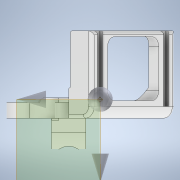
# Autodesk Inventor part: franka_connector
Saved by Autodesk Inventor 2022 (Build 260153000, 153)
## iProperties
Created: 2021-06-02
Part Number: franka_connector
Material: ABS Plastic
Document SubType Name: Modeling
Designer: fraaw
Density: 1.06 g/cm^3
Appearance: Smooth - White
Mass: 33.0638 g
Surface Area: 153.412 cm^2
Volume: 31.1922 cm^3
Author: fraaw
## iProperties of the stored document franka_connector_3DPrint.ipt
Created: 2021-06-08
Part Number: franka_connector_3DPrint
Material: Generic
Document SubType Name: Modeling
Designer: fraaw
Density: 1 g/cm^3
Appearance: Default
Author: fraaw
Autodesk Inventor part; units mm, degrees
note: some values were not read from the file. Chosen so that the rebuilt part matches the saved one: direction of "Hole1".
ref_plane "YZ Plane" through (0, 0, 0) normal (1, 0, 0) x (0, 1, 0)
ref_plane "XZ Plane" through (0, 0, 0) normal (0, 1, 0) x (-1, 0, 0)
ref_plane "XY Plane" through (0, 0, 0) normal (0, 0, 1) x (1, 0, 0)
sketch "Sketch1" plane through (0, 0, 0) normal (0, 1, 0) x (-1, 0, 0)
  line L0 (5, 5) -> (-5, 5) construction
  line L1 (-5, 5) -> (-5, -5) construction
  line L2 (-5, -5) -> (5, -5) construction
  line L3 (5, -5) -> (5, 5) construction
  line L4 (5, 5) -> (-5, -5) construction
  line L5 (-5, 5) -> (5, -5) construction
  line L6 (5, -5) -> (-5, -5) construction
  line L7 (-5, -5) -> (-5, -25)
  line L8 (-5, -25) -> (5, -25)
  line L9 (5, -25) -> (5, -5)
  line L10 (25, 5) -> (5, 5)
  line L11 (25, -5) -> (25, 5)
  line L12 (5, -5) -> (25, -5)
  line L13 (-5, 25) -> (-5, 5)
  line L14 (5, 25) -> (-5, 25)
  line L15 (5, 5) -> (5, 25)
  line L16 (-25, -5) -> (-5, -5)
  line L17 (-25, 5) -> (-25, -5)
  line L18 (-5, 5) -> (-25, 5)
  point P0 (0, 0)
  point P1 (5, -5)
  dimension "d7" = 10
  dimension "d8" = 10
  dimension "d9" = 20
  dimension "d12" = 360
  constraints: 38 end point, 5 equal length, 2 midpoint, 2 perpendicular, 1 horizontal, 29 other
  measures "d7" distance of L1.end L2.end
  measures "d8" distance of L2.end L0.start
  measures "d9" distance of L8.end L2.end
extrude "Extrusion1" add sketch "Sketch1" along normal blind 8
sketch "Sketch2" plane through (0, 8, 0) normal (0, 1, 0) x (1, 0, 0)
  line L0 (5, 25) -> (-5, 25) projected
  circle A0 centre (0, 25) radius 7
  circle A1 centre (-25, 0) radius 7
  circle A2 centre (0, -25) radius 7
  circle A3 centre (25, 0) radius 7
  point P0 (0, 0)
  dimension "d16" = 14
  dimension "d19" = 360
  constraints: 4 centre point, 1 midpoint, 9 other
  measures "d16" diameter of A0
extrude "Base Holes" add sketch "Sketch2" against normal up to surface (8 mm away)
sketch "Sketch3" plane through (0, 8, 0) normal (0, 1, 0) x (1, 0, 0)
  arc A0 (-20.101, 5) -> (-20.101, -5) centre (-25, 0) ccw projected
  point P0 (0, 0)
  point P1 (0, -25)
  point P2 (25, 0)
  point P3 (0, 25)
  dimension "d33" = 360
  constraints: 1 coincident, 5 other
hole "Hole1" at (-25, 8, 0) at (0, 8, 25) at (25, 8, 0) at (0, 8, -25) direction (0, -1, 0) diameter 6.2 depth 8 counterbore diameter 10.1 counterbore depth 4
sketch "Sketch4" plane through (0, 0, 0) normal (0, -1, 0) x (1, 0, 0)
  circle A0 centre (0, -25) radius 3.1 projected
  arc A1 (-5, -20.101) -> (5, -20.101) centre (0, -25) ccw projected
  arc A2 (-5, -20.101) -> (0, -32) centre (0, -25) ccw
  circle A3 centre (-25, 0) radius 3.1 projected
  arc A4 (-20.101, 5) -> (-20.101, -5) centre (-25, 0) ccw projected
  arc A5 (-32, 0) -> (-20.101, -5) centre (-25, 0) ccw
  line L0 (-5, -20.101) -> (-5, -5) projected
  line L1 (-5, -20.101) -> (-5, -5)
  line L2 (-5, -5) -> (-20.101, -5)
  line L3 (-32, 0) -> (-43.1335, 0)
  line L4 (-52.6795, -9.5459) -> (-9.5459, -52.6795)
  line L5 (0, -43.1335) -> (0, -32)
  circle A6 centre (0, 0) radius 44 construction
  line L6 (-43.1335, 0) -> (-52.6795, -9.5459)
  line L7 (-9.5459, -52.6795) -> (0, -43.1335)
  dimension "d49" = 88
  dimension "d50" = 61
  constraints: 14 end point, 8 point on circle, 3 centre point, 3 coincident, 3 perpendicular, 2 equal length, 1 collinear, 1 horizontal, 1 tangent, 1 vertical
  measures "d49" diameter of A6
  measures "d50" distance of L4.start L4.end
extrude "Extrusion3" add sketch "Sketch4" against normal up to surface (8 mm away) contours A1 L5 L7 L4 L6 L3 A4 L2 L0
sketch "Sketch5" plane through (0, 8, 0) normal (0, 1, 0) x (1, 0, 0)
  point P0 (0, 0)
sketch "Sketch6" plane through (0, 8, 0) normal (0, 1, 0) x (1, 0, 0)
  line L0 (-52.6795, 9.5459) -> (-9.5459, 52.6795) projected
  line L1 (-52.6795, 9.5459) -> (-9.5459, 52.6795)
  line L2 (-9.5459, 52.6795) -> (-11.6673, 54.8008)
  line L3 (-11.6673, 54.8008) -> (-54.8008, 11.6673)
  line L4 (-54.8008, 11.6673) -> (-52.6795, 9.5459)
  point P0 (0, 0)
  dimension "d54" = 3
  constraints: 8 end point, 3 equal length, 1 perpendicular
  measures "d54" distance of L3.end L0.start
extrude "Extrusion4" add sketch "Sketch6" against normal blind 45
sketch "Skecth7" plane through (0, 0, 0) normal (0, -1, 0) x (1, 0, 0)
  line L0 (-43.1335, 0) -> (-52.6795, -9.5459) projected
  arc A0 (-43.9916, -0.8581) -> (-0.8581, -43.9916) centre (0, 0) ccw
  line L1 (-9.5459, -52.6795) -> (0, -43.1335) projected
  line L2 (-43.9916, -0.8581) -> (-52.6795, -9.5459)
  line L3 (-43.1335, 0) -> (-54.8008, -11.6673) projected
  line L4 (-52.6795, -9.5459) -> (-9.5459, -52.6795) projected
  line L5 (-31.1127, -31.1127) -> (-9.5459, -52.6795)
  line L6 (-9.5459, -52.6795) -> (-0.8581, -43.9916)
  point P0 (-31.1127, -31.1127)
  dimension "d57" = 44
  constraints: 6 end point, 2 collinear, 2 point on circle, 2 point on line, 1 centre point, 1 coincident, 1 midpoint, 1 perpendicular
  measures "d57" radius of A0
extrude "Extrusion5" add sketch "Skecth7" along normal up to surface (37 mm away)
sketch "Sketch8" plane through (0, -37, 0) normal (0, -1, 0) x (1, 0, 0)
  line L0 (-54.8008, -11.6673) -> (-11.6673, -54.8008) projected
  line L1 (0, 0) -> (-33.234, -33.234) construction
  line L2 (-11.6673, -54.8008) -> (-54.8008, -11.6673) projected
  line L3 (-50.2046, -16.2635) -> (-47.3762, -13.435) construction
  line L4 (-50.2046, -16.2635) -> (-51.6188, -14.8492)
  line L5 (-49.851, -10.9602) -> (-47.3762, -13.435)
  line L6 (-51.6188, -14.8492) -> (-49.851, -10.9602)
  line L7 (-50.2046, -16.2635) -> (-48.7904, -17.6777)
  line L8 (-44.9013, -15.9099) -> (-47.3762, -13.435)
  line L9 (-48.7904, -17.6777) -> (-44.9013, -15.9099)
  line L10 (-16.2635, -50.2046) -> (-13.435, -47.3762) construction
  line L11 (-16.2635, -50.2046) -> (-14.8492, -51.6188)
  line L12 (-10.9602, -49.851) -> (-13.435, -47.3762)
  line L13 (-14.8492, -51.6188) -> (-10.9602, -49.851)
  line L14 (-15.9099, -44.9013) -> (-13.435, -47.3762)
  line L15 (-17.6777, -48.7904) -> (-15.9099, -44.9013)
  line L16 (-16.2635, -50.2046) -> (-17.6777, -48.7904)
  dimension "d81" = 24
  dimension "d82" = 4
  dimension "d83" = 3.5
  dimension "d86" = 2
  constraints: 30 end point, 8 symmetric about line, 3 perpendicular, 2 point on line, 1 midpoint
  measures "d81" distance between parallel lines of L3 L1
  measures "d82" distance from line of L3.end L0
  measures "d83" distance of L5.start L3.end
  measures "d86" distance of L3.start L4.end
extrude "Extrusion6" cut sketch "Sketch8" against normal blind 39
sketch "Sketch18" plane through (0, 8, 0) normal (0, 1, 0) x (1, 0, 0)
  line L0 (8.8, -8.8) -> (-8.8, -8.8)
  line L1 (-8.8, -8.8) -> (-8.8, 8.8)
  line L2 (-8.8, 8.8) -> (8.8, 8.8)
  line L3 (8.8, 8.8) -> (8.8, -8.8)
  line L4 (8.8, -8.8) -> (-8.8, 8.8) construction
  line L5 (-8.8, -8.8) -> (8.8, 8.8) construction
  point P0 (0, 0)
  dimension "d89" = 17.6
  dimension "d90" = 17.6
  constraints: 12 end point, 2 midpoint, 2 parallel, 1 horizontal, 1 perpendicular
  measures "d89" distance of L0.end L1.end
  measures "d90" distance of L1.end L2.end
extrude "Rotator" add sketch "Sketch18" along normal blind 16
fillet "Fillet1" radius 8.8 2 edges at (8.8, 24, 0) (-8.8, 24, 0)
sketch "Sketch9" plane through (8.8, 8, -8.8) normal (0, 0, -1) x (-1, 0, 0)
  arc A0 (17.6, 7.2) -> (0, 7.2) centre (8.8, 7.2) ccw projected
  circle A1 centre (8.8, 7.2) radius 2.4
  point P0 (8.8, -8)
  dimension "d94" = 4.8
  constraints: 1 centre point, 1 coincident
  measures "d94" diameter of A1
extrude "Extrusion8" cut sketch "Sketch9" against normal up to next
sketch "Sketch10" plane through (0, 0, 0) normal (0, -1, 0) x (1, 0, 0)
  line L0 (5, 5) -> (20.101, 5) projected
  arc A0 (14.8825, -5) -> (14.8825, 5) centre (0, 0) ccw
  line L1 (20.101, -5) -> (5, -5) projected
  line L2 (14.8825, 5) -> (5, 5)
  line L3 (5, -5) -> (5, -8.8) projected
  line L4 (14.8825, -5) -> (5, -5)
  arc A1 (5, 14.8825) -> (-5, 14.8825) centre (0, 0) ccw
  line L5 (-5, 14.8825) -> (-5, 5)
  line L6 (5, 14.8825) -> (5, 5)
  arc A2 (-14.8825, 5) -> (-14.8825, -5) centre (0, 0) ccw
  line L7 (-14.8825, -5) -> (-5, -5)
  line L8 (-14.8825, 5) -> (-5, 5)
  arc A3 (-5, -14.8825) -> (5, -14.8825) centre (0, 0) ccw
  line L9 (5, -14.8825) -> (5, -5)
  line L10 (-5, -14.8825) -> (-5, -5)
  dimension "d97" = 15.7
  dimension "d100" = 360
  constraints: 16 end point, 8 point on circle, 4 centre point, 2 point on line, 1 coincident, 1 collinear, 1 horizontal, 33 other
  measures "d97" radius of A0
extrude "Extrusion9" add sketch "Sketch10" along normal blind 2.5
sketch "Sketch21" plane through (0, -2.5, 0) normal (0, -1, 0) x (1, 0, 0)
  circle A0 centre (0, 0) radius 5
  dimension "d104" = 10
  constraints: 1 centre point, 1 coincident
  measures "d104" diameter of A0
extrude "Extrusion10" cut sketch "Sketch21" against normal up to next
chamfer "Chamfer1" distance 8 angle 45 1 edges at (-31.1127, 0, -31.1127)
sketch "Sketch22" plane through (-54.8008, -37, -11.6673) normal (-0.7071068, 0, -0.7071068) x (-0.7071068, 0, 0.7071068)
  line L0 (-8.5, 0) -> (-52.5, 0) projected
  line L1 (-52.5, 39) -> (-51, 39) projected
  line L2 (-8.5, 0) -> (-52.5, 39) construction
  line L3 (-52.5, 0) -> (-8.5, 39) construction
  line L4 (-11.8846, 36) -> (-49.1154, 36)
  line L5 (-49.1154, 36) -> (-49.1154, 3)
  line L6 (-49.1154, 3) -> (-11.8846, 3)
  line L7 (-11.8846, 3) -> (-11.8846, 36)
  line L8 (-11.8846, 36) -> (-49.1154, 3) construction
  line L9 (-49.1154, 36) -> (-11.8846, 3) construction
  point P0 (-30.5, 37)
  point P1 (-30.5, 19.5)
  dimension "d107" = 3
  constraints: 16 end point, 3 midpoint, 3 point on line, 2 parallel, 1 horizontal, 1 perpendicular
  measures "d107" distance between parallel lines of L6 L0
extrude "Extrusion11" cut sketch "Sketch22" against normal up to next
fillet "Fillet3" radius 2.5 4 edges at (0, -2.5, 15.7) (-15.7, -2.5, 0) (0, -2.5, -15.7) (15.7, -2.5, 0)
fillet "Fillet4" radius 5 4 edges at (-14.7592, -1, -41.0853) (-41.0853, -1, -14.7592) (-43.8756, -34, -17.5495) (-17.5495, -34, -43.8756)
sketch "Sketch23" plane through (0, 0, 0) normal (0, 0, 1) x (1, 0, 0)
  line L0 (0, 0) -> (0, -7.1335) projected
  line L1 (0, -7.1335) -> (0, 8) projected
  ellipse E0 centre (0, -20) end of major axis (0, -30) minor radius 7.5
  line L2 (0, 0) -> (7, 0) projected
  point P0 (5, 0)
  dimension "d148" = 10
  dimension "d149" = 7.5
  dimension "d147" = 20
  constraints: 1 point on line, 2 other
  measures "d147" distance from line of L2 point (0, -20)
extrude "Extrusion12" cut sketch "Sketch23" against normal up to next
fillet "Fillet5" radius 6 1 edges at (-33.234, 8, -33.234)
sketch "Sketch28" plane through (0, 8, 0) normal (0, 1, 0) x (1, 0, 0)
  line L0 (-8.8, 8.8) -> (5, 8.8) projected
  line L1 (-8.8, 8.8) -> (-28.9914, 28.9914) construction
  line L2 (-50.5581, 7.4246) -> (-7.4246, 50.5581) projected
  line L3 (-16.2635, 19.0919) -> (-23.3345, 26.163)
  line L4 (-23.3345, 26.163) -> (-26.163, 23.3345)
  line L5 (-26.163, 23.3345) -> (-19.0919, 16.2635)
  line L6 (-19.0919, 16.2635) -> (-16.2635, 19.0919)
  line L7 (-16.2635, 19.0919) -> (-26.163, 23.3345) construction
  line L8 (-23.3345, 26.163) -> (-19.0919, 16.2635) construction
  point P0 (0, 0)
  point P1 (-21.2132, 21.2132)
  dimension "d141" = 10
  dimension "d143" = 4
  dimension "d144" = 11
  constraints: 14 end point, 3 midpoint, 2 parallel, 2 perpendicular, 1 point on line
  measures "d141" distance of L4.end L5.end
  measures "d143" distance of L3.end L4.end
  measures "d144" distance from line of L2 point (-21.213, 21.213)
extrude "Extrusion16" cut sketch "Sketch28" against normal up to next
fillet "Fillet6" radius 2 9 edges at (-53.5582, 6.2427, -10.4246) (-46.8459, 8, -3.7123) (-54.8008, -17.5, -11.6673) (-10.4246, 6.2427, -53.5582) (-3.7123, 8, -46.8459) (-11.6673, -17.5, -54.8008) (-33.234, -37, -33.234) (-53.2098, -37, -13.2583) (-13.2583, -37, -53.2098)
fillet "Fillet7" radius 1 6 edges at (6.9, 8, 8.8) (8.8, 8, 6.9) (-6.9, 8, 8.8) (-8.8, 8, 6.9) (6.9, 8, -8.8) (8.8, 8, -6.9)
sketch "Sketch29" plane through (0, 0, 0) normal (0, -1, 0) x (1, 0, 0)
  line L0 (-19.0919, -16.2635) -> (-16.2635, -19.0919) construction
  line L1 (-17.6777, -17.6777) -> (-24.7487, -24.7487) construction
  line L2 (-19.0919, -16.2635) -> (-26.163, -23.3345) construction
  circle A0 centre (-21.2132, -21.2132) radius 5.3852
  line L3 (-23.3345, -26.163) -> (-26.163, -23.3345) projected
  point P0 (0, 0)
  constraints: 3 midpoint, 2 end point, 1 perpendicular, 3 other
extrude "Extrusion17" cut sketch "Sketch29" along normal mid plane 4
fillet "Fillet8" radius 1 1 edges at (-31.1127, -37, -31.1127)
equation "\"d90\" = d89"
body "Solid1"
